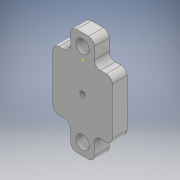
# Autodesk Inventor part: microsoft-lifecam-baseplate
Saved by Autodesk Inventor 2018 (Build 220112000, 112)
## iProperties
Created: 2017-10-09
Part Number: microsoft-lifecam-baseplate
Material: Generic
Document SubType Name: Modeling
Designer: leo2a
Density: 1 g/cm^3
Appearance: Default
Author: leo2a
Autodesk Inventor part; units mm, degrees
ref_plane "YZ Plane" through (0, 0, 0) normal (1, 0, 0) x (0, 1, 0)
ref_plane "XZ Plane" through (0, 0, 0) normal (0, 1, 0) x (-1, 0, 0)
ref_plane "XY Plane" through (0, 0, 0) normal (0, 0, 1) x (1, 0, 0)
sketch "Sketch1" plane through (0, 0, 0) normal (0, 1, 0) x (-1, 0, 0)
  line L0 (-10, 10) -> (-10, -10)
  line L1 (-10, -10) -> (10, -10)
  line L2 (10, -10) -> (10, 10)
  line L3 (10, 10) -> (-10, 10)
  line L4 (-10, 10) -> (10, -10) construction
  line L5 (-10, -10) -> (10, 10) construction
  point P0 (0, 0)
  dimension "d0" = 20
  dimension "d1" = 20
  constraints: 12 end point, 2 midpoint, 2 parallel, 1 perpendicular, 1 vertical
  measures "d0" distance of L0.start L0.end
  measures "d1" distance of L1.end L0.end
extrude "Extrusion1" add sketch "Sketch1" along normal blind 5
sketch "Sketch2" plane through (-10, 0, 10) normal (0, 0, 1) x (1, 0, 0)
  point P0 (10, 0)
sketch "Sketch3" plane through (0, 5, 0) normal (0, 1, 0) x (1, 0, 0)
  point P0 (0, 0)
  point P1 (0, 0)
  constraints: 1 coincident
hole "Hole1" at (0, 5, 0) direction (0, -1, 0) diameter 1.8 end through all counterbore diameter 7.5 counterbore depth 3 clearance for "Socket Head Cap Screw" size "M1.6" standard "Ansi Metric M Profile"
sketch "Sketch4" plane through (-10, 0, 10) normal (0, 0, 1) x (1, 0, 0)
  line L0 (10, 0) -> (10, 1.5)
  line L1 (14, 3) -> (14, 0)
  line L2 (14, 0) -> (6, 0)
  line L3 (6, 0) -> (6, 3)
  line L4 (6, 3) -> (14, 3)
  line L5 (14, 3) -> (6, 0) construction
  line L6 (14, 0) -> (6, 3) construction
  dimension "d11" = 8
  constraints: 14 end point, 3 parallel, 2 midpoint, 1 perpendicular, 1 vertical
  measures "d11" distance of L1.end L2.end
extrude "Extrusion2" add sketch "Sketch4" along normal blind 8
mirror "Mirror1" about plane through (0, 0, 0) normal (0, 0, 1) of "Extrusion2"
sketch "Sketch5" plane through (0, 5, 0) normal (0, 1, 0) x (1, 0, 0)
  line L0 (0, 0) -> (0, -14)
  line L1 (0, 0) -> (0, 14)
  dimension "d14" = 14
  dimension "d15" = 14
  constraints: 4 end point, 2 coincident, 2 vertical
  measures "d14" distance of L0.start L0.end
  measures "d15" distance of L0.start L1.end
hole "Hole2" at (0, 5, 14) at (0, 5, -14) direction (0, -1, 0) diameter 4.5 end through all clearance for "Socket Head Cap Screw" size "M4" standard "Ansi Metric M Profile"
fillet "Fillet1" radius 2 12 edges at (4, 1.5, 10) (4, 1.5, 18) (10, 2.5, 10) (10, 2.5, -10) (4, 1.5, -10) (4, 1.5, -18) (-4, 1.5, -18) (-4, 1.5, -10) (-10, 2.5, -10) (-10, 2.5, 10) (-4, 1.5, 10) (-4, 1.5, 18)
move faces "Move1" translate (0, 2, 0) faces at (0, 3, 10.5833)
move faces "Move2" translate (0, 2, 0) faces at (3.4661, 2, -17.3603) (4.5339, 2, -10.6397) (0, 3, -10.8742)
body "Solid1"
